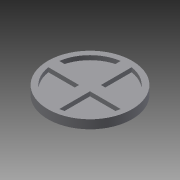
# Autodesk Inventor part: regalPlasticsDisk
Saved by Autodesk Inventor 2014 (Build 180170000, 170)
## iProperties
Created: 2014-02-10
Part Number: regalPlasticsDisk
Material: Generic
Document SubType Name: Modeling
Designer: clang
Density: 1 g/cm^3
Appearance: Default
Author: clang
Autodesk Inventor part; units mm, degrees
ref_plane "YZ Plane" through (0, 0, 0) normal (1, 0, 0) x (0, 1, 0)
ref_plane "XZ Plane" through (0, 0, 0) normal (0, 1, 0) x (-1, 0, 0)
ref_plane "XY Plane" through (0, 0, 0) normal (0, 0, 1) x (1, 0, 0)
sketch "Sketch1" plane through (0, 0, 0) normal (0, 1, 0) x (-1, 0, 0)
  circle A0 centre (0, 0) radius 123.0248
  arc A1 (16.0001, -105.822) -> (105.8221, -15.9999) centre (0, 0) ccw
  line L0 (16.0001, -105.822) -> (16.0001, -16.0002)
  line L1 (16.0001, -16.0002) -> (105.8221, -15.9999)
  arc A2 (105.8221, 15.9999) -> (16.0001, 105.822) centre (0, 0) ccw
  line L2 (16.0001, 105.822) -> (16.0001, 16.0002)
  line L3 (16.0001, 16.0002) -> (105.8221, 15.9999)
  arc A3 (-105.8221, -15.9999) -> (-16.0001, -105.822) centre (0, 0) ccw
  line L4 (-16.0001, -105.822) -> (-16.0001, -16.0002)
  line L5 (-16.0001, -16.0002) -> (-105.8221, -15.9999)
  line L6 (-16.0001, 16.0002) -> (-105.8221, 15.9999)
  line L7 (-16.0001, 105.822) -> (-16.0001, 16.0002)
  arc A4 (-16.0001, 105.822) -> (-105.8221, 15.9999) centre (0, 0) ccw
  line L8 (16.0001, -16.0002) -> (107.9989, -16.0002)
  line L9 (16.0001, -16.0002) -> (16.0001, -107.999)
  line L10 (16.0001, -16.0002) -> (105.5859, -16.0002) construction
  arc A5 (16.0001, -107.999) -> (107.9989, -16.0002) centre (9.6855, -9.6856) ccw
  line L11 (75.678, -75.6779) -> (158.1368, -75.6779) construction
  line L12 (75.678, -75.6779) -> (278.878, -75.6779) construction
  line L13 (16.0001, -135.3558) -> (16.0001, -16.0002)
  dimension "d1" = 107.0248
  dimension "d4" = 89.8218
  dimension "d12" = 91.9988
  dimension "d13" = 91.9988
  dimension "d19" = 119.3556
  constraints: 28 end point, 11 point on circle, 6 centre point, 3 horizontal, 3 perpendicular, 2 coincident
  measures "d1" radius of A1
  measures "d4" distance of L0.start L0.end
  measures "d12" distance of L0.end L8.end
  measures "d13" distance of L0.end L9.end
  measures "d19" distance of L13.start L0.end
sketch "Sketch2" plane through (0, 0, 0) normal (0, 1, 0) x (-1, 0, 0)
  circle A0 centre (0, 0) radius 123.0248
  arc A1 (16.0001, -105.822) -> (105.8221, -15.9999) centre (0, 0) ccw
  line L0 (0, 0) -> (105.8221, -15.9999) construction
  line L1 (0, 0) -> (107.0248, 0) construction
  line L2 (0, 0) -> (16.0001, -105.822) construction
  line L3 (16.0001, -105.822) -> (16.0001, -16.0002)
  line L4 (16.0001, -105.822) -> (105.8219, -105.822) construction
  line L5 (16.0001, -16.0002) -> (105.8221, -15.9999)
  line L6 (16.0001, 16.0002) -> (105.8221, 15.9999)
  line L7 (16.0001, 105.822) -> (16.0001, 16.0002)
  arc A2 (105.8221, 15.9999) -> (16.0001, 105.822) centre (0, 0) ccw
  line L8 (-16.0001, 16.0002) -> (-105.8221, 15.9999)
  line L9 (-16.0001, 105.822) -> (-16.0001, 16.0002)
  arc A3 (-16.0001, 105.822) -> (-105.8221, 15.9999) centre (0, 0) ccw
  arc A4 (-105.8221, -15.9999) -> (-16.0001, -105.822) centre (0, 0) ccw
  line L10 (-16.0001, -16.0002) -> (-105.8221, -15.9999)
  line L11 (-16.0001, -105.822) -> (-16.0001, -16.0002)
  dimension "d6" = 107.0248
  dimension "d7" = 89.8218
  constraints: 24 end point, 8 point on circle, 5 centre point, 3 symmetric about line, 2 coincident, 2 equal length, 2 horizontal, 1 perpendicular, 1 other
  measures "d6" radius of A1
  measures "d7" distance of L2.end L3.end
extrude "Extrusion1" add sketch "Sketch2" along normal blind 25.4
extrude "Extrusion2" add sketch "Sketch1" along normal blind 12.7 contours L0 L1 A1 | L3 L2 A2 | L5 L4 A3 | L6 A4 L7
body "Solid1"
